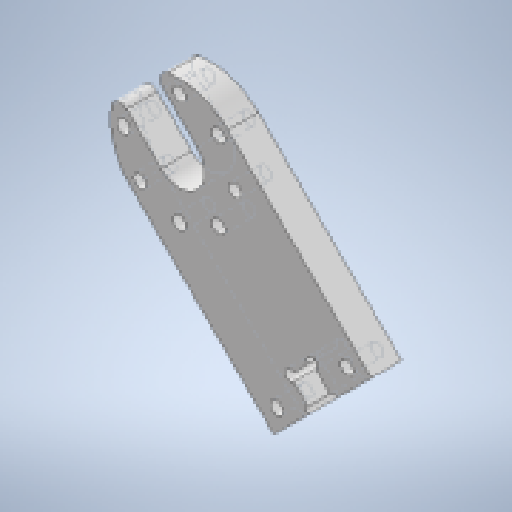
# Autodesk Inventor part: ankle
Saved by Autodesk Inventor 2024 (Build 280153000, 153)
## iProperties
Created: 2024-09-17
Part Number: ankle
Material: 일반
Document SubType Name: Modeling
Designer: Eungang
Density: 1 g/cm^3
Appearance: 기본값
Author: Eungang
Autodesk Inventor part; units mm, degrees
ref_plane "YZ Plane" through (0, 0, 0) normal (1, 0, 0) x (0, 1, 0)
ref_plane "XZ Plane" through (0, 0, 0) normal (0, 1, 0) x (-1, 0, 0)
ref_plane "XY Plane" through (0, 0, 0) normal (0, 0, 1) x (1, 0, 0)
sketch "스케치1" plane through (0, 0, 0) normal (0, 0, 1) x (1, 0, 0)
  line L0 (25.7798, -6.5464) -> (-2.5045, 21.7378) projected
  arc A0 (-2.5045, 21.7378) -> (-14.369, 25.5341) centre (-12.1212, 12.1212) ccw projected
  arc A1 (-14.369, 25.5341) -> (-15.3443, 22.4861) centre (-14.0715, 23.7589) ccw projected
  line L1 (-15.3443, 22.4861) -> (-8.5503, 15.6921) projected
  arc A2 (-15.6921, 8.5503) -> (-8.5503, 15.6921) centre (-12.1212, 12.1212) ccw projected
  line L2 (-15.6921, 8.5503) -> (-22.4861, 15.3443) projected
  arc A3 (-22.4861, 15.3443) -> (-25.5341, 14.369) centre (-23.7589, 14.0715) ccw projected
  arc A4 (-25.5341, 14.369) -> (-21.7378, 2.5045) centre (-12.1212, 12.1212) ccw projected
  line L3 (-21.7378, 2.5045) -> (6.5464, -25.7798) projected
  line L4 (6.5464, -25.7798) -> (13.3347, -18.9915) projected
  arc A5 (13.2675, -17.6516) -> (13.3347, -18.9915) centre (14.0418, -18.2844) ccw projected
  line L5 (13.2675, -17.6516) -> (10.432, -14.8161) projected
  arc A6 (10.432, -13.2675) -> (10.432, -14.8161) centre (9.7991, -14.0418) ccw projected
  line L6 (10.432, -13.2675) -> (13.2675, -10.432) projected
  arc A7 (14.8161, -10.432) -> (13.2675, -10.432) centre (14.0418, -9.7991) ccw projected
  line L7 (14.8161, -10.432) -> (17.6516, -13.2675) projected
  arc A8 (18.9915, -13.3347) -> (17.6516, -13.2675) centre (18.2844, -14.0418) ccw projected
  line L8 (18.9915, -13.3347) -> (25.7798, -6.5464) projected
  circle A9 centre (20.9714, -7.1121) radius 1.25 projected
  circle A10 centre (-19.8993, 4.343) radius 1.2812 projected
  circle A11 centre (-23.1212, 12.1212) radius 1.2812 projected
  circle A12 centre (-4.343, 4.343) radius 1.2812 projected
  circle A13 centre (-1.1212, 12.1212) radius 1.2812 projected
  circle A14 centre (-12.1212, 1.1212) radius 1.2812 projected
  circle A15 centre (-4.343, 19.8993) radius 1.2812 projected
  circle A16 centre (-12.1212, 23.1212) radius 1.2812 projected
  circle A17 centre (7.1121, -20.9714) radius 1.25 projected
  line L9 (10.432, -14.8161) -> (13.2675, -17.6516)
  line L10 (14.8161, -10.432) -> (17.6516, -13.2675)
  point P0 (0, 0)
  constraints: 4 end point, 1 parallel
extrude "돌출1" add sketch "스케치1" against normal blind 6
